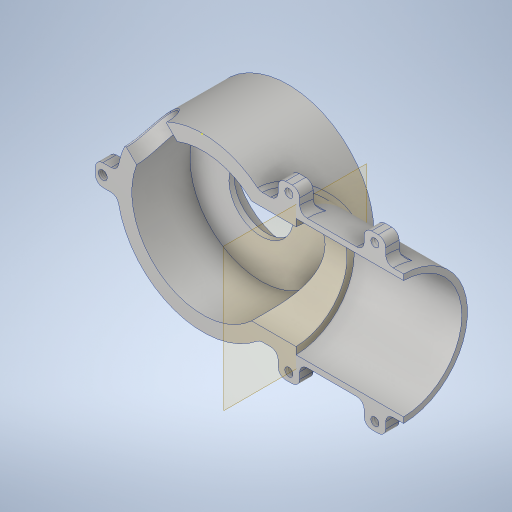
# Autodesk Inventor part: AR-001B
Saved by Autodesk Inventor 2023.4 (Build 274418000, 418)
## iProperties
Created: 2025-01-22
Part Number: AR-001B
Material: Aluminum 6061
Document SubType Name: Modeling
Designer: jmcintyr
Density: 2.7 g/cm^3
Appearance: Aluminum - Flat
Mass: 424.302 g
Surface Area: 617.506 cm^2
Volume: 157.149 cm^3
Author: jmcintyr
Autodesk Inventor part; units mm, degrees
sketch "Sketch1" plane through (0, 0, 0) normal (0, 0, 1) x (1, 0, 0)
  circle A0 centre (0, 0) radius 38.1
  dimension "d0" = 76.2
  constraints: 1 centre point, 1 coincident
  measures "d0" diameter of A0
extrude "Extrusion1" add sketch "Sketch1" along normal mid plane 76.2
ref_plane "Work Plane1" through (88.9, 0, 0) normal (1, 0, 0) x (0, 1, 0)
sketch "Sketch2" plane through (88.9, 0, 0) normal (1, 0, 0) x (0, 1, 0)
  circle A0 centre (0, 0) radius 26.162
  circle A1 centre (0, 0) radius 28.702
  dimension "d4" = 52.324
  dimension "d5" = 2.54
  constraints: 2 centre point, 1 coincident
  measures "d4" diameter of A0
  measures "d5" radial gap between concentric circles of A0 A1
extrude "Extrusion2" add sketch "Sketch2" against normal up to next
sketch "Sketch3" plane through (88.9, 0, 0) normal (1, 0, 0) x (0, 1, 0)
  circle A0 centre (0, 0) radius 26.162 projected
extrude "Extrusion3" cut sketch "Sketch3" against normal blind 83.82
sketch "Sketch4" plane through (0, 0, 38.1) normal (0, 0, 1) x (1, 0, 0)
  point P0 (0, 0)
  point P1 (0, 0)
  constraints: 1 coincident
hole "Hole1" at (0, 0, 38.1) direction (0, 0, -1) diameter 28.575 depth 41.275 tip angle 118 counterbore diameter 47.625 counterbore depth 9.525
ref_plane "Work Plane2" through (0, 0, 38.1) normal (0, 0, 1) x (1, 0, 0)
ref_plane "Work Plane3" through (-47.625, 0, 0) normal (1, 0, 0) x (0, 1, 0)
sketch "Sketch7" plane through (-47.625, 0, 0) normal (1, 0, 0) x (0, 1, 0)
  line L0 (4.7625, 6.35) -> (-4.7625, 6.35)
  line L1 (-4.7625, 6.35) -> (-4.7625, -6.35)
  line L2 (-4.7625, -6.35) -> (4.7625, -6.35)
  line L3 (4.7625, -6.35) -> (4.7625, 6.35)
  line L4 (4.7625, 6.35) -> (-4.7625, -6.35) construction
  line L5 (-4.7625, 6.35) -> (4.7625, -6.35) construction
  point P0 (0, 0)
  dimension "d28" = 9.525
  dimension "d29" = 12.7
  constraints: 12 end point, 2 midpoint, 2 parallel, 1 horizontal, 1 perpendicular
  measures "d28" distance of L2.end L1.end
  measures "d29" distance of L1.end L0.end
extrude "Extrusion5" add sketch "Sketch7" along normal up to next
sketch "Sketch8" plane through (0, 0, -38.1) normal (0, 0, -1) x (-1, 0, 0)
  point P0 (0, 0)
  point P1 (0, 0)
  constraints: 1 coincident
hole "Hole2" at (0, 0, -38.1) direction (0, 0, 1) diameter 28.575 end up to surface counterbore diameter 47.625 counterbore depth 9.525
ref_plane "Work Plane8" through (41.275, 0, 0) normal (1, 0, 0) x (0, 0, -1)
sketch "Sketch22" plane through (41.275, 0, 0) normal (1, 0, 0) x (0, 0, -1)
  circle A0 centre (0, 0) radius 26.162 projected
  circle A1 centre (0, 0) radius 28.702 projected
  circle A2 centre (0, 0) radius 22.987
  dimension "d114" = 3.175
  constraints: 1 centre point, 1 coincident
  measures "d114" radial gap between concentric circles of A2 A0
extrude "Extrusion14" add sketch "Sketch22" against normal up to surface (36.195 mm away) contours A0
sketch "Sketch9" plane through (0, 0, 0) normal (0, 0, 1) x (1, 0, 0)
  circle A0 centre (0, 0) radius 31.5139
  constraints: 1 centre point, 1 coincident
extrude "Extrusion6" cut sketch "Sketch9" along normal mid plane 52.3875
sketch "Sketch10" plane through (0, 0, 38.1) normal (0, 0, 1) x (1, 0, 0)
  circle A0 centre (0, 0) radius 38.1 projected
  circle A1 centre (0, 0) radius 34.8488 construction
  line L0 (17.4625, -30.1625) -> (-17.4625, -30.1625) construction
  line L1 (-17.4625, -30.1625) -> (-17.4625, 30.1625) construction
  line L2 (-17.4625, 30.1625) -> (17.4625, 30.1625) construction
  line L3 (17.4625, 30.1625) -> (17.4625, -30.1625) construction
  line L4 (17.4625, -30.1625) -> (-17.4625, 30.1625) construction
  line L5 (-17.4625, -30.1625) -> (17.4625, 30.1625) construction
  dimension "d43" = 69.6976
  dimension "d44" = 34.925
  dimension "d45" = 60.325
  constraints: 12 end point, 5 coincident, 2 midpoint, 2 parallel, 1 centre point, 1 horizontal, 1 perpendicular
  measures "d43" diameter of A1
  measures "d44" distance of L1.end L2.end
  measures "d45" distance of L0.end L1.end
hole "Hole3" at (-17.4625, 30.1625, 38.1) at (17.4625, 30.1625, 38.1) at (17.4625, -30.1625, 38.1) at (-17.4625, -30.1625, 38.1) direction (0, 0, -1) diameter 4.3434 depth 25.4 tip angle 118 thread size "12-24 UNC" class "2B" standard "ANSI Unified Screw Threads"
fillet "Fillet4" radius 3.302 6 edges at (-38.1, 0, 6.35) (-37.8012, -4.7625, 0) (-38.1, 0, -6.35) (-37.8012, 4.7625, 0) (-47.625, -4.7625, 0) (-47.625, 4.7625, 0)
mirror "Mirror2" about plane through (0, 0, 0) normal (0, 0, 1) of "Hole3"
sketch "Sketch13" plane through (-47.625, -1.4605, -6.35) normal (0, 0, -1) x (-1, 0, 0)
  line L0 (-88.9, 26.8402) -> (-136.525, 26.8402) construction
  line L1 (-136.525, 26.8402) -> (-136.525, 29.4513) construction
  line L2 (-136.525, 29.4513) -> (-73.4732, 29.4513) construction
  arc A0 (-10.2548, 8.8818) -> (-7.016, 6.223) centre (-7.016, 9.525) ccw construction
  line L3 (-7.016, 6.223) -> (-6.4978, 6.223) construction
  arc A1 (-6.4978, -3.302) -> (-6.4978, 6.223) centre (-47.625, 1.4605) ccw construction
  line L4 (-3.302, -3.302) -> (-6.4978, -3.302) construction
  arc A2 (-3.302, -3.302) -> (0, 0) centre (-3.302, 0) ccw construction
  line L5 (0, 2.921) -> (0, 0) construction
  arc A3 (0, 2.921) -> (-3.302, 6.223) centre (-3.302, 2.921) ccw construction
  line L6 (-6.4978, 6.223) -> (-3.302, 6.223) construction
  line L7 (-136.525, -23.9192) -> (-88.9, -23.9192) construction
  line L8 (-136.525, -26.5303) -> (-136.525, -23.9192) construction
  line L9 (-73.4732, -26.5303) -> (-136.525, -26.5303) construction
  line L10 (-6.4978, -3.302) -> (-7.016, -3.302) construction
  arc A4 (-7.016, -3.302) -> (-10.2548, -5.9608) centre (-7.016, -6.604) ccw construction
  line L11 (-3.302, 0) -> (-3.302, 2.921) construction
  arc A5 (-10.2548, 8.8818) -> (-73.4732, 29.4513) centre (-47.625, 1.4605) ccw projected
  arc A6 (-73.4732, -26.5303) -> (-10.2548, -5.9608) centre (-47.625, 1.4605) ccw projected
  arc A7 (-70.0982, -20.632) -> (-70.0982, 23.553) centre (-47.625, 1.4605) ccw projected
  line L12 (-70.0982, 23.553) -> (-88.9, 23.553) projected
  line L13 (-88.9, 23.553) -> (-88.9, 26.8402) projected
  line L14 (-88.9, -20.632) -> (-70.0982, -20.632) projected
  line L15 (-88.9, -23.9192) -> (-88.9, -20.632) projected
  point P0 (-3.302, 1.4605)
  constraints: 2 end point, 1 midpoint, 1 vertical
hole "Hole5" at (-44.323, 0, -6.35) direction (0, 0, 1) diameter 3.9624 end through all thread size "10-32 UNF" class "2B" standard "ANSI Unified Screw Threads"
sketch "Sketch14" plane through (0, 0, 38.1) normal (0, 0, 1) x (1, 0, 0)
  circle A0 centre (0, 0) radius 38.1 construction
  circle A1 centre (17.4625, -30.1625) radius 2.1717 construction
  circle A2 centre (-17.4625, 30.1625) radius 2.1717 construction
  circle A3 centre (17.4625, 30.1625) radius 2.1717 construction
  circle A4 centre (-17.4625, -30.1625) radius 2.1717 construction
  circle A5 centre (0, 0) radius 23.8125 construction
  circle A6 centre (0, 0) radius 38.1 construction
  line L0 (-26.9408, 26.9408) -> (0, 0) construction
  line L1 (0, 0) -> (-38.1, 0) construction
  dimension "d77" = 45
  constraints: 4 end point, 2 point on circle, 1 horizontal, 1 other
  measures "d77" angle of L1 L0
ref_plane "Work Plane4" through (-26.9408, 26.9408, 38.1) normal (-0.7071068, 0.7071068, 0) x (-0.7071068, -0.7071068, 0)
sketch "Sketch15" plane through (-26.9408, 26.9408, 38.1) normal (-0.7071068, 0.7071068, 0) x (-0.7071068, -0.7071068, 0)
  line L0 (0, -76.2) -> (0, 0) construction
  circle A0 centre (0, -38.1) radius 12.7
  dimension "d78" = 25.4
  constraints: 1 centre point, 1 coincident, 1 midpoint
  measures "d78" diameter of A0
extrude "Extrusion8" cut sketch "Sketch15" against normal up to surface round surface about axis through (0, 0, 0) along (0, 0, 1) radius 31.5139 far side no
fillet "Fillet5" radius 0.508 3 edges at (-32.9047, 19.2066, -8.2141) (-32.9047, 19.2066, 8.2141) (-16.4197, 34.3803, -0.0099)
ref_plane "Work Plane5" through (0, 38.1, 0) normal (0, 1, 0) x (-1, 0, 0)
sketch "Sketch16" plane through (0, 38.1, 0) normal (0, 1, 0) x (-1, 0, 0)
  line L0 (-33.3375, -6.35) -> (-42.8625, -6.35)
  line L1 (-42.8625, -6.35) -> (-42.8625, 6.35)
  line L2 (-42.8625, 6.35) -> (-33.3375, 6.35)
  line L3 (-33.3375, 6.35) -> (-33.3375, -6.35)
  line L4 (-33.3375, -6.35) -> (-42.8625, 6.35) construction
  line L5 (-42.8625, -6.35) -> (-33.3375, 6.35) construction
  line L6 (0, -38.1) -> (0, 38.1) construction
  line L7 (-71.4375, -6.35) -> (-80.9625, -6.35)
  line L8 (-80.9625, -6.35) -> (-80.9625, 6.35)
  line L9 (-80.9625, 6.35) -> (-71.4375, 6.35)
  line L10 (-71.4375, 6.35) -> (-71.4375, -6.35)
  line L11 (-71.4375, -6.35) -> (-80.9625, 6.35) construction
  line L12 (-80.9625, -6.35) -> (-71.4375, 6.35) construction
  point P0 (0, 0)
  point P1 (-38.1, 0)
  point P2 (0, 0)
  point P3 (-76.2, 0)
  dimension "d84" = 9.525
  dimension "d85" = 12.7
  dimension "d86" = 38.1
  dimension "d96" = 38.1
  constraints: 24 end point, 5 midpoint, 4 parallel, 2 equal length, 2 horizontal, 2 horizontal alignment, 2 perpendicular
  measures "d84" distance of L1.end L2.end
  measures "d85" distance of L0.end L1.end
  measures "d86" distance of point (0, 0) point (-38.1, 0)
  measures "d96" distance of point (-76.2, 0) point (-38.1, 0)
extrude "Extrusion9" add sketch "Sketch16" against normal up to next
ref_plane "Work Plane6" through (0, -38.1, 0) normal (0, 1, 0) x (-1, 0, 0)
sketch "Sketch17" plane through (0, -38.1, 0) normal (0, 1, 0) x (-1, 0, 0)
  line L0 (-42.8625, -6.35) -> (-33.3375, -6.35)
  line L1 (-33.3375, -6.35) -> (-33.3375, 6.35)
  line L2 (-33.3375, 6.35) -> (-42.8625, 6.35)
  line L3 (-42.8625, 6.35) -> (-42.8625, -6.35)
  line L4 (-42.8625, -6.35) -> (-33.3375, 6.35) construction
  line L5 (-33.3375, -6.35) -> (-42.8625, 6.35) construction
  line L6 (-80.9625, -6.35) -> (-71.4375, -6.35)
  line L7 (-71.4375, -6.35) -> (-71.4375, 6.35)
  line L8 (-71.4375, 6.35) -> (-80.9625, 6.35)
  line L9 (-80.9625, 6.35) -> (-80.9625, -6.35)
  line L10 (-80.9625, -6.35) -> (-71.4375, 6.35) construction
  line L11 (-71.4375, -6.35) -> (-80.9625, 6.35) construction
  point P0 (0, 0)
  point P1 (-38.1, 0)
  point P2 (-76.2, 0)
  dimension "d90" = 9.525
  dimension "d91" = 12.7
  dimension "d92" = 38.1
  dimension "d95" = 38.1
  constraints: 24 end point, 4 midpoint, 4 parallel, 2 equal length, 2 horizontal, 2 horizontal alignment, 2 perpendicular
  measures "d90" distance of L2.end L1.end
  measures "d91" distance of L1.end L0.end
  measures "d92" distance of point (0, 0) point (-38.1, 0)
  measures "d95" distance of point (-38.1, 0) point (-76.2, 0)
extrude "Extrusion10" add sketch "Sketch17" along normal up to next
fillet "Fillet6" radius 3.302 32 edges at (33.3375, 38.1, 0) (42.8625, 38.1, 0) (71.4375, 38.1, 0) (80.9625, 38.1, 0) (80.9625, -38.1, 0) (42.8625, -38.1, 0) (33.3375, -38.1, 0) (71.4375, -38.1, 0) (33.3375, -28.702, 0) (38.1, -27.9908, -6.35) (42.8625, -28.702, 0) (38.1, -27.9908, 6.35) (76.2, -27.9908, 6.35) (80.9625, -28.702, 0) (76.2, -27.9908, -6.35) (71.4375, -28.702, 0) (38.1, 27.9908, -6.35) (42.8625, 28.5236, -3.1949) (42.8625, 28.5236, 3.1949) (33.3375, 28.5236, -3.1949) (33.3375, 28.5236, 3.1949) (71.4375, 28.5236, -3.1949) (71.4375, 28.5236, 3.1949) (76.2, 27.9908, -6.35) (80.9625, 28.5236, -3.1949) (80.9625, 28.5236, 3.1949) (76.2, 27.9908, 6.35) (31.2425, 21.8063, 18.6625) (31.2425, 21.8064, -18.6624) (31.2425, -21.8063, -18.6625) (31.2415, -21.8077, 18.6609) (38.1, 27.9908, 6.35)
sketch "Sketch18" plane through (36.6395, 38.1, 6.35) normal (0, 0, 1) x (1, 0, 0)
  line L0 (-49.7449, -9.4404) -> (-54.1835, -5.0017) construction
  arc A0 (-11.7726, -9.234) -> (-53.9699, -4.1697) centre (-36.6395, -38.1) ccw construction
  line L1 (-9.4365, -10.1092) -> (-6.604, -10.1092) construction
  line L2 (-3.302, -6.7323) -> (-3.302, -3.302) construction
  arc A1 (0, 0) -> (-3.302, -3.302) centre (0, -3.302) ccw construction
  line L3 (0, 0) -> (2.921, 0) construction
  arc A2 (6.223, -3.302) -> (2.921, 0) centre (2.921, -3.302) ccw construction
  line L4 (6.223, -3.302) -> (6.223, -6.7323) construction
  line L5 (-3.4097, -7.5862) -> (6.3307, -7.5862) construction
  arc A3 (-14.1663, -16.0075) -> (-49.7449, -9.4404) centre (-36.6395, -38.1) ccw construction
  line L6 (52.2605, -12.7203) -> (4.6355, -12.7203) construction
  line L7 (52.2605, -10.1092) -> (52.2605, -12.7203) construction
  line L8 (47.625, -10.1092) -> (52.2605, -10.1092) construction
  line L9 (34.6903, -7.5862) -> (44.4307, -7.5862) construction
  line L10 (9.525, -10.1092) -> (31.496, -10.1092) construction
  line L11 (44.323, -3.302) -> (44.323, -6.7323) construction
  arc A4 (44.323, -3.302) -> (41.021, 0) centre (41.021, -3.302) ccw construction
  line L12 (38.1, 0) -> (41.021, 0) construction
  arc A5 (38.1, 0) -> (34.798, -3.302) centre (38.1, -3.302) ccw construction
  line L13 (34.798, -6.7323) -> (34.798, -3.302) construction
  circle A6 centre (-80.9625, -38.1) radius 1.9812 construction
  line L14 (-77.2485, -42.8625) -> (-77.7667, -42.8625) construction
  line L15 (-77.7667, -42.8625) -> (-80.9625, -42.8625) construction
  arc A7 (-84.2645, -39.5605) -> (-80.9625, -42.8625) centre (-80.9625, -39.5605) ccw construction
  line L16 (-84.2645, -39.5605) -> (-84.2645, -36.6395) construction
  arc A8 (-80.9625, -33.3375) -> (-84.2645, -36.6395) centre (-80.9625, -36.6395) ccw construction
  line L17 (-80.9625, -33.3375) -> (-77.7667, -33.3375) construction
  line L18 (-77.7667, -33.3375) -> (-77.2485, -33.3375) construction
  arc A9 (-77.2485, -33.3375) -> (-74.0097, -30.6787) centre (-77.2485, -30.0355) ccw construction
  arc A10 (-70.5698, -20.7696) -> (-74.0097, -30.6787) centre (-36.6395, -38.1) ccw construction
  line L19 (-69.7378, -20.556) -> (-65.2991, -24.9946) construction
  arc A11 (-65.2991, -24.9946) -> (-14.1663, -60.1925) centre (-36.6395, -38.1) ccw construction
  line L20 (4.6355, -63.4797) -> (52.2605, -63.4797) construction
  line L21 (52.2605, -63.4797) -> (52.2605, -66.0908) construction
  line L22 (52.2605, -66.0908) -> (47.625, -66.0908) construction
  line L23 (44.323, -69.4677) -> (44.323, -72.898) construction
  arc A12 (41.021, -76.2) -> (44.323, -72.898) centre (41.021, -72.898) ccw construction
  line L24 (41.021, -76.2) -> (38.1, -76.2) construction
  arc A13 (34.798, -72.898) -> (38.1, -76.2) centre (38.1, -72.898) ccw construction
  line L25 (34.798, -72.898) -> (34.798, -69.4677) construction
  line L26 (31.496, -66.0908) -> (9.525, -66.0908) construction
  line L27 (6.223, -69.4677) -> (6.223, -72.898) construction
  arc A14 (2.921, -76.2) -> (6.223, -72.898) centre (2.921, -72.898) ccw construction
  line L28 (2.921, -76.2) -> (0, -76.2) construction
  arc A15 (-3.302, -72.898) -> (0, -76.2) centre (0, -72.898) ccw construction
  line L29 (-3.302, -72.898) -> (-3.302, -69.4677) construction
  line L30 (-6.604, -66.0908) -> (-9.4365, -66.0908) construction
  arc A16 (-74.0097, -45.5213) -> (-11.7726, -66.966) centre (-36.6395, -38.1) ccw construction
  arc A17 (-74.0097, -45.5213) -> (-77.2485, -42.8625) centre (-77.2485, -46.1645) ccw construction
  arc A18 (-77.7667, -33.3375) -> (-77.7667, -42.8625) centre (-36.6395, -38.1) ccw construction
  line L31 (44.4307, -68.6138) -> (34.6903, -68.6138) construction
  line L32 (6.3307, -68.6138) -> (-3.4097, -68.6138) construction
  line L33 (0, -3.302) -> (2.921, -3.302) construction
  line L34 (38.1, -3.302) -> (41.021, -3.302) construction
  line L35 (6.3307, -7.5862) -> (-3.4097, -7.5862) construction
  line L36 (1.4605, -7.5862) -> (1.4605, 0) construction
  line L37 (2.921, 0) -> (0, 0) construction
  line L38 (-3.4097, -68.6138) -> (6.3307, -68.6138) construction
  line L39 (1.4605, -68.6138) -> (1.4605, -76.2) construction
  line L40 (0, -76.2) -> (2.921, -76.2) construction
  line L41 (4.6355, -16.0075) -> (-14.1663, -16.0075) projected
  line L42 (4.6355, -12.7203) -> (4.6355, -16.0075) projected
  line L43 (-14.1663, -60.1925) -> (4.6355, -60.1925) projected
  line L44 (4.6355, -60.1925) -> (4.6355, -63.4797) projected
  point P0 (1.4605, -3.7931)
  point P1 (39.5605, -3.7931)
  point P2 (39.5605, -72.4069)
  point P3 (1.4605, -72.4069)
  point P4 (1.4605, -3.302)
  point P5 (1.4605, -3.7931)
  point P6 (39.5605, -3.302)
  point P7 (1.4605, -72.4069)
  point P8 (-17.958, -63.4797)
  constraints: 8 end point, 8 midpoint, 4 vertical alignment, 3 coincident, 2 horizontal, 2 horizontal alignment, 20 other
hole "Hole6" at (38.1, 34.3069, 6.35) at (76.2, 34.3069, 6.35) at (76.2, -34.3069, 6.35) at (38.1, -34.3069, 6.35) direction (0, 0, -1) diameter 3.683 end through all thread size "10-24 UNC" class "2B" standard "ANSI Unified Screw Threads"
ref_plane "Work Plane7" through (38.1, 0, 0) normal (1, 0, 0) x (0, 0, -1)
sketch "Sketch19" plane through (38.1, 0, 0) normal (1, 0, 0) x (0, 0, -1)
  arc A0 (-8.6562, 27.3656) -> (-24.7521, 14.5307) centre (0, 0) ccw construction
  arc A1 (-8.6562, 27.3656) -> (-6.35, 30.5138) centre (-9.652, 30.5138) ccw construction
  line L0 (-6.35, 30.5138) -> (-6.35, 32.4654) construction
  line L1 (6.35, 32.4654) -> (6.35, 30.5138) construction
  arc A2 (6.35, 30.5138) -> (8.6562, 27.3656) centre (9.652, 30.5138) ccw construction
  arc A3 (24.7521, 14.5307) -> (8.6562, 27.3656) centre (0, 0) ccw construction
  arc A4 (8.6562, -27.3656) -> (24.7521, -14.5307) centre (0, 0) ccw construction
  arc A5 (8.6562, -27.3656) -> (6.35, -30.5138) centre (9.652, -30.5138) ccw construction
  line L2 (6.35, -30.5138) -> (6.35, -32.4654) construction
  line L3 (-6.35, -32.4654) -> (-6.35, -30.5138) construction
  arc A6 (-6.35, -30.5138) -> (-8.6562, -27.3656) centre (-9.652, -30.5138) ccw construction
  arc A7 (-24.7521, -14.5307) -> (-8.6562, -27.3656) centre (0, 0) ccw construction
  line L4 (-32.004, 0) -> (-38.1, 0) construction
  line L5 (38.1, 0) -> (32.004, 0) construction
  circle A8 centre (0, 0) radius 26.162
  circle A9 centre (0, 0) radius 23.622
  line L6 (6.35, 36.1484) -> (-6.35, 36.1484) projected
  line L7 (-6.35, 36.1484) -> (-6.35, 38.1) projected
  line L8 (-6.35, 38.1) -> (6.35, 38.1) projected
  line L9 (6.35, 38.1) -> (6.35, 36.1484) projected
  line L10 (-6.35, -36.1484) -> (6.35, -36.1484) projected
  line L11 (6.35, -36.1484) -> (6.35, -38.1) projected
  line L12 (6.35, -38.1) -> (-6.35, -38.1) projected
  line L13 (-6.35, -38.1) -> (-6.35, -36.1484) projected
  line L14 (-6.35, 32.4654) -> (6.35, 32.4654) projected
  line L15 (6.35, -32.4654) -> (-6.35, -32.4654) projected
  circle A10 centre (0, 0) radius 22.987 projected
  dimension "d106" = 2.54
  constraints: 2 centre point, 1 coincident, 4 other
  measures "d106" radial gap between concentric circles of A8 A9
extrude "Extrusion11" [suppressed]
split body "Split1" result two bodies by plane through (0, 0, 0) normal (0, 0, 1) first body at (19.3029, 32.267, 14.4746)
sketch "Sketch20" plane through (0, 0, 0) normal (0, 0, 1) x (1, 0, 0)
  line L0 (30.0355, -28.702) -> (26.2654, -28.702) construction
  arc A0 (-37.3702, -7.4213) -> (24.1706, -29.4515) centre (0, 0) ccw construction
  arc A1 (-37.3702, -7.4213) -> (-40.609, -4.7625) centre (-40.609, -8.0645) ccw construction
  line L1 (-40.609, -4.7625) -> (-44.323, -4.7625) construction
  arc A2 (-47.625, -1.4605) -> (-44.323, -4.7625) centre (-44.323, -1.4605) ccw construction
  line L2 (-47.625, -1.4605) -> (-47.625, 1.4605) construction
  arc A3 (-44.323, 4.7625) -> (-47.625, 1.4605) centre (-44.323, 1.4605) ccw construction
  line L3 (-44.323, 4.7625) -> (-40.609, 4.7625) construction
  arc A4 (-40.609, 4.7625) -> (-37.3702, 7.4213) centre (-40.609, 8.0645) ccw construction
  arc A5 (-34.6888, 15.7574) -> (-37.3702, 7.4213) centre (0, 0) ccw construction
  line L4 (-33.8671, 15.9066) -> (-29.3743, 11.4138) construction
  arc A6 (-29.3743, 11.4138) -> (21.5574, -22.987) centre (0, 0) ccw construction
  line L5 (41.275, -26.162) -> (88.9, -26.162) construction
  line L6 (88.9, -26.162) -> (88.9, -28.702) construction
  line L7 (88.9, -28.702) -> (84.2645, -28.702) construction
  arc A7 (84.2645, -28.702) -> (80.9625, -32.004) centre (84.2645, -32.004) ccw construction
  line L8 (80.9625, -32.004) -> (80.9625, -34.798) construction
  arc A8 (77.6605, -38.1) -> (80.9625, -34.798) centre (77.6605, -34.798) ccw construction
  line L9 (77.6605, -38.1) -> (74.7395, -38.1) construction
  arc A9 (71.4375, -34.798) -> (74.7395, -38.1) centre (74.7395, -34.798) ccw construction
  line L10 (71.4375, -34.798) -> (71.4375, -32.004) construction
  arc A10 (71.4375, -32.004) -> (68.1355, -28.702) centre (68.1355, -32.004) ccw construction
  line L11 (68.1355, -28.702) -> (46.1645, -28.702) construction
  arc A11 (46.1645, -28.702) -> (42.8625, -32.004) centre (46.1645, -32.004) ccw construction
  line L12 (42.8625, -32.004) -> (42.8625, -34.798) construction
  arc A12 (39.5605, -38.1) -> (42.8625, -34.798) centre (39.5605, -34.798) ccw construction
  line L13 (39.5605, -38.1) -> (36.6395, -38.1) construction
  arc A13 (33.3375, -34.798) -> (36.6395, -38.1) centre (36.6395, -34.798) ccw construction
  line L14 (33.3375, -34.798) -> (33.3375, -32.004) construction
  arc A14 (33.3375, -32.004) -> (30.0355, -28.702) centre (30.0355, -32.004) ccw construction
  circle A15 centre (-44.323, 0) radius 1.9812 construction
  circle A16 centre (38.1, -34.3069) radius 1.8415 construction
  circle A17 centre (76.2, -34.3069) radius 1.8415 construction
  circle A18 centre (38.1, 34.3069) radius 1.8415 construction
  circle A19 centre (76.2, 34.3069) radius 1.8415 construction
  arc A20 (80.9625, 34.798) -> (77.6605, 38.1) centre (77.6605, 34.798) ccw construction
  line L15 (80.9625, 34.798) -> (80.9625, 32.004) construction
  arc A21 (80.9625, 32.004) -> (84.2645, 28.702) centre (84.2645, 32.004) ccw construction
  line L16 (84.2645, 28.702) -> (88.9, 28.702) construction
  line L17 (88.9, 28.702) -> (88.9, 26.162) construction
  line L18 (88.9, 26.162) -> (41.275, 26.162) construction
  arc A22 (21.5574, 22.987) -> (-11.4138, 29.3743) centre (0, 0) ccw construction
  line L19 (-11.4138, 29.3743) -> (-15.9066, 33.8671) construction
  arc A23 (24.1706, 29.4515) -> (-15.7574, 34.6888) centre (0, 0) ccw construction
  line L20 (26.2654, 28.702) -> (30.0355, 28.702) construction
  arc A24 (30.0355, 28.702) -> (33.3375, 32.004) centre (30.0355, 32.004) ccw construction
  line L21 (33.3375, 32.004) -> (33.3375, 34.798) construction
  arc A25 (36.6395, 38.1) -> (33.3375, 34.798) centre (36.6395, 34.798) ccw construction
  line L22 (36.6395, 38.1) -> (39.5605, 38.1) construction
  arc A26 (42.8625, 34.798) -> (39.5605, 38.1) centre (39.5605, 34.798) ccw construction
  line L23 (42.8625, 34.798) -> (42.8625, 32.004) construction
  arc A27 (42.8625, 32.004) -> (46.1645, 28.702) centre (46.1645, 32.004) ccw construction
  line L24 (46.1645, 28.702) -> (68.1355, 28.702) construction
  arc A28 (68.1355, 28.702) -> (71.4375, 32.004) centre (68.1355, 32.004) ccw construction
  line L25 (71.4375, 32.004) -> (71.4375, 34.798) construction
  arc A29 (74.7395, 38.1) -> (71.4375, 34.798) centre (74.7395, 34.798) ccw construction
  line L26 (74.7395, 38.1) -> (77.6605, 38.1) construction
  line L27 (-47.625, 38.1) -> (88.9, 38.1)
  line L28 (88.9, 38.1) -> (88.9, -38.1)
  line L29 (88.9, -38.1) -> (-47.625, -38.1)
  line L30 (-47.625, -38.1) -> (-47.625, 38.1)
  line L31 (41.275, 26.162) -> (41.275, 22.987) projected
  line L32 (41.275, 22.987) -> (21.5574, 22.987) projected
  line L33 (21.5574, -22.987) -> (41.275, -22.987) projected
  line L34 (41.275, -22.987) -> (41.275, -26.162) projected
  point P0 (76.2, 38.1)
  point P1 (-47.625, 0)
  point P2 (38.1, -38.1)
  constraints: 8 end point, 4 midpoint, 3 point on line, 2 parallel, 1 horizontal, 1 perpendicular, 4 other
extrude "Extrusion12" cut sketch "Sketch20" against normal blind 0.381 bodies 3
sketch "Sketch21" plane through (0, 0, 0) normal (0, 0, 1) x (1, 0, 0)
  line L0 (88.9, 38.1) -> (-47.625, 38.1)
  line L1 (-47.625, 38.1) -> (-47.625, -38.1)
  line L2 (-47.625, -38.1) -> (88.9, -38.1)
  line L3 (88.9, -38.1) -> (88.9, 38.1)
  line L4 (30.0355, -28.702) -> (26.2654, -28.702) construction
  arc A0 (-37.3702, -7.4213) -> (24.1706, -29.4515) centre (0, 0) ccw construction
  arc A1 (-37.3702, -7.4213) -> (-40.609, -4.7625) centre (-40.609, -8.0645) ccw construction
  line L5 (-40.609, -4.7625) -> (-44.323, -4.7625) construction
  arc A2 (-47.625, -1.4605) -> (-44.323, -4.7625) centre (-44.323, -1.4605) ccw construction
  line L6 (-47.625, -1.4605) -> (-47.625, 1.4605) construction
  arc A3 (-44.323, 4.7625) -> (-47.625, 1.4605) centre (-44.323, 1.4605) ccw construction
  line L7 (-44.323, 4.7625) -> (-40.609, 4.7625) construction
  arc A4 (-40.609, 4.7625) -> (-37.3702, 7.4213) centre (-40.609, 8.0645) ccw construction
  arc A5 (-34.6888, 15.7574) -> (-37.3702, 7.4213) centre (0, 0) ccw construction
  line L8 (-33.8671, 15.9066) -> (-29.3743, 11.4138) construction
  arc A6 (-29.3743, 11.4138) -> (21.5574, -22.987) centre (0, 0) ccw construction
  line L9 (41.275, -26.162) -> (88.9, -26.162) construction
  line L10 (88.9, -26.162) -> (88.9, -28.702) construction
  line L11 (88.9, -28.702) -> (84.2645, -28.702) construction
  arc A7 (84.2645, -28.702) -> (80.9625, -32.004) centre (84.2645, -32.004) ccw construction
  line L12 (80.9625, -32.004) -> (80.9625, -34.798) construction
  arc A8 (77.6605, -38.1) -> (80.9625, -34.798) centre (77.6605, -34.798) ccw construction
  line L13 (77.6605, -38.1) -> (74.7395, -38.1) construction
  arc A9 (71.4375, -34.798) -> (74.7395, -38.1) centre (74.7395, -34.798) ccw construction
  line L14 (71.4375, -34.798) -> (71.4375, -32.004) construction
  arc A10 (71.4375, -32.004) -> (68.1355, -28.702) centre (68.1355, -32.004) ccw construction
  line L15 (68.1355, -28.702) -> (46.1645, -28.702) construction
  arc A11 (46.1645, -28.702) -> (42.8625, -32.004) centre (46.1645, -32.004) ccw construction
  line L16 (42.8625, -32.004) -> (42.8625, -34.798) construction
  arc A12 (39.5605, -38.1) -> (42.8625, -34.798) centre (39.5605, -34.798) ccw construction
  line L17 (39.5605, -38.1) -> (36.6395, -38.1) construction
  arc A13 (33.3375, -34.798) -> (36.6395, -38.1) centre (36.6395, -34.798) ccw construction
  line L18 (33.3375, -34.798) -> (33.3375, -32.004) construction
  arc A14 (33.3375, -32.004) -> (30.0355, -28.702) centre (30.0355, -32.004) ccw construction
  circle A15 centre (-44.323, 0) radius 1.9812 construction
  circle A16 centre (38.1, -34.3069) radius 1.8415 construction
  circle A17 centre (76.2, -34.3069) radius 1.8415 construction
  circle A18 centre (38.1, 34.3069) radius 1.8415 construction
  circle A19 centre (76.2, 34.3069) radius 1.8415 construction
  arc A20 (80.9625, 34.798) -> (77.6605, 38.1) centre (77.6605, 34.798) ccw construction
  line L19 (80.9625, 34.798) -> (80.9625, 32.004) construction
  arc A21 (80.9625, 32.004) -> (84.2645, 28.702) centre (84.2645, 32.004) ccw construction
  line L20 (84.2645, 28.702) -> (88.9, 28.702) construction
  line L21 (88.9, 28.702) -> (88.9, 26.162) construction
  line L22 (88.9, 26.162) -> (41.275, 26.162) construction
  arc A22 (21.5574, 22.987) -> (-11.4138, 29.3743) centre (0, 0) ccw construction
  line L23 (-11.4138, 29.3743) -> (-15.9066, 33.8671) construction
  arc A23 (24.1706, 29.4515) -> (-15.7574, 34.6888) centre (0, 0) ccw construction
  line L24 (26.2654, 28.702) -> (30.0355, 28.702) construction
  arc A24 (30.0355, 28.702) -> (33.3375, 32.004) centre (30.0355, 32.004) ccw construction
  line L25 (33.3375, 32.004) -> (33.3375, 34.798) construction
  arc A25 (36.6395, 38.1) -> (33.3375, 34.798) centre (36.6395, 34.798) ccw construction
  line L26 (36.6395, 38.1) -> (39.5605, 38.1) construction
  arc A26 (42.8625, 34.798) -> (39.5605, 38.1) centre (39.5605, 34.798) ccw construction
  line L27 (42.8625, 34.798) -> (42.8625, 32.004) construction
  arc A27 (42.8625, 32.004) -> (46.1645, 28.702) centre (46.1645, 32.004) ccw construction
  line L28 (46.1645, 28.702) -> (68.1355, 28.702) construction
  arc A28 (68.1355, 28.702) -> (71.4375, 32.004) centre (68.1355, 32.004) ccw construction
  line L29 (71.4375, 32.004) -> (71.4375, 34.798) construction
  arc A29 (74.7395, 38.1) -> (71.4375, 34.798) centre (74.7395, 34.798) ccw construction
  line L30 (74.7395, 38.1) -> (77.6605, 38.1) construction
  line L31 (41.275, 26.162) -> (41.275, 22.987) projected
  line L32 (41.275, 22.987) -> (21.5574, 22.987) projected
  line L33 (21.5574, -22.987) -> (41.275, -22.987) projected
  line L34 (41.275, -22.987) -> (41.275, -26.162) projected
  point P0 (76.2, 38.1)
  point P1 (-47.625, 0)
  point P2 (88.9, -27.432)
  point P3 (38.1, -38.1)
  constraints: 8 end point, 5 midpoint, 3 point on line, 2 parallel, 1 horizontal, 1 perpendicular, 4 other
extrude "Extrusion13" cut sketch "Sketch21" along normal blind 0.381 bodies 2
sketch "Sketch23" plane through (0, 38.1, 0) normal (0, 1, 0) x (1, 0, 0)
  point P0 (0, 0)
body "Solid2"
body "Solid3"
